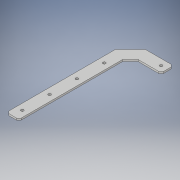
# Autodesk Inventor part: gnd
Saved by Autodesk Inventor 2019 (Build 230136000, 136)
## iProperties
Created: 2019-07-08
Part Number: gnd
Material: Ogólny
Document SubType Name: Modeling
Designer: Kurat
Density: 1 g/cm^3
Appearance: Domyślna
Author: Kurat
Autodesk Inventor part; units mm, degrees
ref_plane "YZ Plane" through (0, 0, 0) normal (1, 0, 0) x (0, 1, 0)
ref_plane "XZ Plane" through (0, 0, 0) normal (0, 1, 0) x (-1, 0, 0)
ref_plane "XY Plane" through (0, 0, 0) normal (0, 0, 1) x (1, 0, 0)
sketch "Szkic1" plane through (0, 0, 0) normal (0, 1, 0) x (-1, 0, 0)
  line L0 (0, -1.91) -> (0, -62.23)
  line L1 (0, -62.23) -> (-8.8883, -71.1183)
  line L2 (0, -62.23) -> (12.57, -62.23) construction
  line L3 (-8.8883, -71.1183) -> (-24.1183, -71.1183)
  line L4 (-26.0283, -69.2083) -> (-26.0283, -64.1383)
  line L5 (-24.1183, -62.2283) -> (-12.6883, -62.2283)
  line L6 (-12.6883, -62.2283) -> (-8.877, -58.417)
  line L7 (-12.6883, -62.2283) -> (-7.2983, -62.2283) construction
  line L8 (-8.877, -58.417) -> (-8.877, -1.91)
  line L9 (-6.967, 0) -> (-1.91, 0)
  line L10 (-1.91, 0) -> (0, -1.91)
  line L11 (-8.877, -1.91) -> (-6.967, 0)
  line L12 (-26.0283, -64.1383) -> (-24.1183, -62.2283)
  line L13 (-26.0283, -69.2083) -> (-24.1183, -71.1183)
  line L14 (-26.0283, -66.6733) -> (-15.6934, -66.6733)
  circle A0 centre (-21.5783, -66.6733) radius 0.75
  line L15 (-4.4385, 0) -> (-4.4385, -63.1833)
  circle A1 centre (-4.4385, -6.35) radius 0.75
  circle A2 centre (-4.4385, -21.59) radius 0.75
  circle A3 centre (-4.4385, -36.83) radius 0.75
  circle A4 centre (-4.4385, -52.07) radius 0.75
  line L16 (-1, -61.8158) -> (-1, -2.3242)
  line L17 (-1, -2.3242) -> (-2.3242, -1)
  line L18 (-2.3242, -1) -> (-6.5528, -1)
  line L19 (-6.5528, -1) -> (-7.877, -2.3242)
  line L20 (-7.877, -2.3242) -> (-7.877, -58.8312)
  line L21 (-7.877, -58.8312) -> (-12.2741, -63.2283)
  line L22 (-12.2741, -63.2283) -> (-23.7041, -63.2283)
  line L23 (-23.7041, -63.2283) -> (-25.0283, -64.5525)
  line L24 (-25.0283, -64.5525) -> (-25.0283, -68.7941)
  line L25 (-25.0283, -68.7941) -> (-23.7041, -70.1183)
  line L26 (-23.7041, -70.1183) -> (-9.3025, -70.1183)
  line L27 (-9.3025, -70.1183) -> (-1, -61.8158)
  point P0 (0, 0)
  point P1 (-26.0283, -71.1183)
  point P2 (-26.0283, -62.2283)
  point P3 (-8.877, 0)
  dimension "d0" = 62.23
  dimension "d1" = 135
  dimension "d2" = 12.57
  dimension "d3" = 17.14
  dimension "d4" = 8.89
  dimension "d5" = 13.34
  dimension "d6" = 45
  dimension "d7" = 5.39
  dimension "d8" = 1.91
  dimension "d9" = 1.91
  dimension "d10" = 1.91
  dimension "d11" = 1.91
  dimension "d12" = 1.91
  dimension "d13" = 1.91
  dimension "d14" = 1.91
  dimension "d15" = 1.91
  dimension "d16" = 1.5
  dimension "d17" = 4.45
  dimension "d18" = 1.5
  dimension "d19" = 6.35
  dimension "d22" = 15.24
  dimension "d27" = 19.048
  dimension "d28" = 1
  dimension "d31" = 45.72
  constraints: 56 end point, 10 point on line, 5 centre point, 5 horizontal, 5 vertical, 2 equal length, 2 midpoint, 2 perpendicular, 17 other
  measures "d0" distance of point (0, 0) L0.end
  measures "d1" angle of L1 L2
  measures "d2" distance of L0.end L1.end
  measures "d3" distance of L1.end point (-26.028, -71.118)
  measures "d4" distance of point (-26.028, -71.118) point (-26.028, -62.228)
  measures "d5" distance of point (-26.028, -62.228) L5.end
  measures "d6" angle of L7 L6
  measures "d7" distance of L5.end L6.end
  measures "d8" distance of L9.end point (0, 0)
  measures "d9" distance of L0.start point (0, 0)
  measures "d10" distance of L8.end point (-8.877, 0)
  measures "d11" distance of L9.start point (-8.877, 0)
  measures "d12" distance of L4.end point (-26.028, -62.228)
  measures "d13" distance of L5.start point (-26.028, -62.228)
  measures "d14" distance of L4.start point (-26.028, -71.118)
  measures "d15" distance of L3.end point (-26.028, -71.118)
  measures "d16" diameter of A0
  measures "d17" distance of L14.start A0.centre
  measures "d18" diameter of A1
  measures "d19" distance of L15.start A1.centre
  measures "d22" distance of A1.centre A2.centre
  measures "d28" distance between parallel lines of L0 L16
  measures "d31" distance of A4.centre A1.centre
extrude "Wyciągnięcie proste1" add sketch "Szkic1" along normal blind 1 contours L18 L17 L16 L27 L26 L25 L24 L23 L22 L21 L20 L19
equation "\"d9\" = d8"
equation "\"d10\" = d8"
equation "\"d11\" = d10"
equation "\"d12\" = d8"
equation "\"d13\" = d12"
equation "\"d14\" = d8"
equation "\"d15\" = d14"
